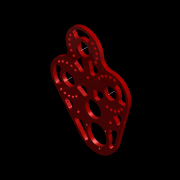
# Autodesk Inventor part: Part2
Saved by Autodesk Inventor 2014 SP1 (Build 180222100, 222)
## iProperties
Created: 2014-01-05
Part Number: Part2
Material: Aluminum 6061
Document SubType Name: Modeling
Designer: Rauhul Varma
Density: 2.71 g/cm^3
Appearance: Red
Mass: 189.365 g
Surface Area: 361.578 cm^2
Volume: 69.8764 cm^3
Author: Rauhul Varma
Autodesk Inventor part; units mm, degrees
note: some values were not read from the file. Chosen so that the rebuilt part matches the saved one: direction of "Hole3".
ref_plane "YZ Plane" through (0, 0, 0) normal (1, 0, 0) x (0, 1, 0)
ref_plane "XZ Plane" through (0, 0, 0) normal (0, 1, 0) x (-1, 0, 0)
sketch "Main Outline" plane through (0, 0, 0) normal (0, 0, 1) x (1, 0, 0)
  line L0 (0, 0) -> (304.8, 0) construction
  line L1 (304.8, 0) -> (304.8, 50.8) construction
  line L2 (304.8, 50.8) -> (0, 50.8) construction
  line L3 (0, 50.8) -> (0, 0) construction
  line L4 (0, 50.8) -> (0, 53.34) construction
  line L5 (0, 53.34) -> (304.8, 53.34) construction
  line L6 (304.8, 53.34) -> (304.8, 50.8) construction
  circle A0 centre (152.4, 23.8125) radius 17.4625 construction
  line L7 (152.4, 23.8125) -> (152.4, 0) construction
  circle A1 centre (152.4, 23.8125) radius 27.94 construction
  circle A2 centre (152.4, 23.8125) radius 21.59 construction
  line L8 (152.4, 23.8125) -> (144.7964, 60.3681) construction
  circle A3 centre (144.7964, 60.3681) radius 15.24 construction
  circle A4 centre (144.7964, 60.3681) radius 8.89 construction
  circle A5 centre (144.7964, 60.3681) radius 14.2875 construction
  arc A6 (164.6591, 71.8014) -> (129.0153, 43.7486) centre (144.7964, 60.3681) ccw construction
  circle A7 centre (98.8106, 85.598) radius 32.258 construction
  circle A8 centre (126.6733, 147.4971) radius 32.258 construction
  circle A9 centre (176.9075, 101.8424) radius 32.258 construction
  circle A10 centre (144.7964, 60.3681) radius 11.1125 construction
  circle A11 centre (152.4, 23.8125) radius 49.53 construction
  line L9 (144.7964, 60.3681) -> (126.6733, 147.4971) construction
  line L10 (144.7964, 60.3681) -> (98.8106, 85.598) construction
  line L11 (98.8106, 85.598) -> (176.9075, 101.8424) construction
  line L12 (176.9075, 101.8424) -> (144.7964, 60.3681) construction
  circle A12 centre (98.8106, 85.598) radius 9.5493 construction
  arc A13 (174.9629, 111.1915) -> (185.6989, 98.1139) centre (176.9075, 101.8424) ccw construction
  circle A14 centre (126.6733, 147.4971) radius 9.5493 construction
  line L13 (96.8659, 94.9472) -> (174.9629, 111.1915) construction
  line L14 (185.6989, 98.1139) -> (165.8956, 51.4198) construction
  line L15 (92.2351, 78.6732) -> (129.0153, 43.7486) construction
  line L16 (174.9629, 111.1915) -> (176.9075, 101.8424) construction
  line L17 (176.9075, 101.8424) -> (185.6989, 98.1139) construction
  arc A15 (185.6989, 98.1139) -> (174.9629, 111.1915) centre (176.9075, 101.8424) ccw construction
  arc A16 (165.8956, 51.4198) -> (164.6591, 71.8014) centre (144.7964, 60.3681) ccw construction
  arc A17 (129.0153, 43.7486) -> (165.8956, 51.4198) centre (144.7964, 60.3681) ccw construction
  circle A18 centre (126.6086, 147.808) radius 32.258 construction
  circle A19 centre (126.544, 148.1188) radius 32.258 construction
  circle A20 centre (126.4793, 148.4297) radius 32.258 construction
  line L18 (126.6733, 147.4971) -> (126.4793, 148.4297) construction
  circle A21 centre (126.738, 147.1863) radius 32.258 construction
  circle A22 centre (117.4622, 43.2997) radius 9.525 construction
  circle A23 centre (176.6694, 55.615) radius 9.525 construction
  line L19 (152.4, 23.8125) -> (117.4622, 43.2997) construction
  line L20 (152.4, 23.8125) -> (176.6694, 55.615) construction
  line L21 (117.4622, 43.2997) -> (98.8106, 85.598) construction
  line L22 (176.6694, 55.615) -> (176.9075, 101.8424) construction
  circle A24 centre (135.1821, 106.5897) radius 7.9375 construction
  line L23 (135.6243, 150.8242) -> (166.2787, 68.353) construction
  circle A25 centre (152.4, 23.8125) radius 29.845 construction
  line L24 (117.1381, 146.979) -> (121.9118, 59.1246) construction
  circle A26 centre (99.0889, 85.4453) radius 32.258 construction
  circle A27 centre (97.9755, 86.0562) radius 32.258 construction
  line L25 (97.9755, 86.0562) -> (98.8106, 85.598) construction
  circle A28 centre (98.2538, 85.9034) radius 32.258 construction
  circle A29 centre (98.5322, 85.7507) radius 32.258 construction
  circle A30 centre (152.4, 23.8125) radius 29.845 construction
  circle A31 centre (122.555, 23.8125) radius 6.35 construction
  circle A32 centre (179.7696, 35.7133) radius 6.35 construction
  line L26 (122.555, 23.8125) -> (152.4, 23.8125) construction
  line L27 (152.4, 23.8125) -> (182.245, 23.8125) construction
  circle A33 centre (182.245, 23.8125) radius 6.35 construction
  circle A34 centre (125.0304, 11.9117) radius 6.35 construction
  circle A35 centre (150.4199, 33.3321) radius 39.5684 construction
  line L28 (72.9795, 65.6655) -> (119.7593, 8.3204) construction
  circle A36 centre (177.4906, 102.5955) radius 32.258 construction
  line L29 (176.9075, 101.8424) -> (177.4906, 102.5955) construction
  circle A37 centre (177.2963, 102.3445) radius 32.258 construction
  circle A38 centre (177.1019, 102.0934) radius 32.258 construction
  circle A39 centre (176.7131, 101.5913) radius 32.258 construction
  line L30 (188.5109, 22.6209) -> (208.5442, 93.8632) construction
  circle A40 centre (135.1821, 106.5897) radius 9.5727 construction
  arc A41 (86.8202, 116.3239) -> (96.3065, 136.4856) centre (81.3304, 131.2195) ccw construction
  arc A42 (158.9123, 149.5077) -> (175.6513, 134.801) centre (174.7462, 150.6502) ccw construction
  line L31 (126.4793, 148.4297) -> (126.9966, 145.9429) construction
  line L32 (116.5322, 146.3607) -> (117.0495, 143.8739) construction
  line L33 (136.9437, 148.0119) -> (136.4264, 150.4987) construction
  arc A43 (136.4264, 150.4987) -> (116.5322, 146.3607) centre (126.4793, 148.4297) ccw construction
  arc A44 (117.0495, 143.8739) -> (136.9437, 148.0119) centre (126.9966, 145.9429) ccw construction
  line L34 (177.4906, 102.5955) -> (175.9357, 100.5871) construction
  line L35 (169.4571, 108.8154) -> (167.9021, 106.807) construction
  line L36 (183.9692, 94.3672) -> (185.5242, 96.3756) construction
  arc A45 (185.5242, 96.3756) -> (169.4571, 108.8154) centre (177.4906, 102.5955) ccw construction
  arc A46 (167.9021, 106.807) -> (183.9692, 94.3672) centre (175.9357, 100.5871) ccw construction
  line L37 (97.9755, 86.0562) -> (100.2023, 84.8344) construction
  line L38 (93.0884, 77.1487) -> (95.3153, 75.927) construction
  line L39 (105.0894, 93.7418) -> (102.8625, 94.9636) construction
  arc A47 (102.8625, 94.9636) -> (93.0884, 77.1487) centre (97.9755, 86.0562) ccw construction
  arc A48 (95.3153, 75.927) -> (105.0894, 93.7418) centre (100.2023, 84.8344) ccw construction
  circle A49 centre (117.4622, 43.2997) radius 3.9687 construction
  circle A50 centre (176.6694, 55.615) radius 3.9687 construction
  line L40 (152.4, 23.8125) -> (158.4777, -5.4071) construction
  arc A51 (80.1751, 59.3139) -> (79.0947, 58.1692) centre (79.7097, 58.6709) ccw construction
  arc A52 (205.9254, 84.5503) -> (204.4781, 85.1692) centre (205.1613, 84.7652) ccw construction
  circle A53 centre (152.4, 23.8125) radius 14.224 construction
  circle A54 centre (135.1821, 106.5897) radius 3.9687 construction
  circle A55 centre (156.538, 3.9183) radius 6.35 construction
  circle A56 centre (156.538, 3.9183) radius 2.0828 construction
  circle A57 centre (152.4, 23.8125) radius 20.32 construction
  line L41 (133.1021, 30.1759) -> (152.4, 23.8125) construction
  line L42 (152.4, 23.8125) -> (167.5599, 37.3432) construction
  circle A58 centre (167.5599, 37.3432) radius 2.0828 construction
  circle A59 centre (167.5599, 37.3432) radius 3.9687 construction
  circle A60 centre (133.1021, 30.1759) radius 2.0828 construction
  circle A61 centre (133.1021, 30.1759) radius 3.9688 construction
  point P0 (126.738, 147.1863)
  point P1 (176.7131, 101.5913)
  dimension "d18" = 99.06
  dimension "d58" = 64.516
  dimension "d86" = 64.516
  dimension "d0" = 304.8
  dimension "d1" = 50.8
  dimension "d2" = 2.54
  dimension "d3" = 34.925
  dimension "d4" = 23.8125
  dimension "d5" = 152.4
  dimension "d6" = 55.88
  dimension "d7" = 43.18
  dimension "d8" = 37.338
  dimension "d10" = 30.48
  dimension "d11" = 17.78
  dimension "d12" = 28.575
  dimension "d13" = 45.8366
  dimension "d14" = 64.516
  dimension "d15" = 64.516
  dimension "d16" = 64.516
  dimension "d17" = 22.225
  dimension "d19" = 52.4523
  dimension "d20" = 88.9939
  dimension "d21" = 19.0986
  dimension "d22" = 19.0986
  dimension "d23" = 19.0986
  dimension "d30" = 124.732
  dimension "d40" = 64.516
  dimension "d41" = 64.516
  dimension "d42" = 64.516
  dimension "d43" = 0.9525
  dimension "d44" = 0.3175
  dimension "d45" = 0.635
  dimension "d46" = 64.516
  dimension "d47" = 0.3175
  dimension "d48" = 19.05
  dimension "d49" = 19.05
  dimension "d50" = 40.005
  dimension "d51" = 40.005
  dimension "d52" = 46.228
  dimension "d54" = 46.228
  dimension "d55" = 15.875
  dimension "d56" = 41.4655
  dimension "d57" = 59.69
  dimension "d59" = 64.516
  dimension "d60" = 64.516
  dimension "d61" = 64.516
  dimension "d62" = 0.3175
  dimension "d63" = 0.3175
  dimension "d64" = 0.635
  dimension "d65" = 0.9525
  dimension "d73" = 12.7
  dimension "d74" = 12.7
  dimension "d76" = 59.69
  dimension "d78" = 12.7
  dimension "d79" = 12.7
  dimension "d80" = 64.516
  dimension "d81" = 0.9525
  dimension "d82" = 64.516
  dimension "d83" = 64.516
  dimension "d84" = 0.3175
  dimension "d85" = 0.635
  dimension "d88" = 0.3175
  dimension "d89" = 31.75
  dimension "d90" = 31.75
  dimension "d94" = 1.5875
  dimension "d95" = 20.32
  dimension "d96" = 1.5875
  constraints: 92 end point, 59 centre point, 54 point on circle, 38 tangent, 26 coincident, 16 point on line, 9 collinear, 6 parallel, 4 midpoint, 4 perpendicular, 3 symmetric about line, 2 horizontal, 13 other
  measures "d0" distance of L2.end L1.end
  measures "d1" distance of L1.end L0.end
  measures "d2" distance of L2.end L4.end
  measures "d3" diameter of A0
  measures "d4" distance of L7.start L7.end
  measures "d5" distance between parallel lines of L3 L7
  measures "d6" diameter of A1
  measures "d7" diameter of A2
  measures "d8" distance of L8.start L8.end
  measures "d10" diameter of A3
  measures "d11" diameter of A4
  measures "d12" diameter of A5
  measures "d13" diameter of A6
  measures "d14" diameter of A7
  measures "d15" diameter of A8
  measures "d16" diameter of A9
  measures "d17" diameter of A10
  measures "d19" distance of L9.start L10.end
  measures "d20" distance of L9.start L9.end
  measures "d21" diameter of A12
  measures "d22" diameter of A13
  measures "d23" diameter of A14
  measures "d30" angle of L17 L16
  measures "d40" diameter of A18
  measures "d41" diameter of A19
  measures "d42" diameter of A20
  measures "d43" distance of L18.end L9.end
  measures "d44" distance of A18.centre L9.end
  measures "d45" distance of A19.centre L9.end
  measures "d46" diameter of A21
  measures "d47" distance of L9.end A21.centre
  measures "d48" diameter of A22
  measures "d49" diameter of A23
  measures "d50" distance of L19.start L19.end
  measures "d51" distance of L19.start L20.end
  measures "d52" distance of L19.end L21.end
  measures "d54" distance of L20.end L16.end
  measures "d55" diameter of A24
  measures "d56" distance of A21.centre A24.centre
  measures "d57" diameter of A25
  measures "d59" diameter of A27
  measures "d60" diameter of A28
  measures "d61" diameter of A29
  measures "d62" distance of point (99.089, 85.445) L10.end
  measures "d63" distance of L10.end A29.centre
  measures "d64" distance of L10.end A28.centre
  measures "d65" distance of L25.start L10.end
  measures "d73" diameter of A31
  measures "d74" diameter of A32
  measures "d76" diameter of A30
  measures "d78" diameter of A33
  measures "d79" diameter of A34
  measures "d80" diameter of A36
  measures "d81" distance of L29.start L29.end
  measures "d82" diameter of A37
  measures "d83" diameter of A38
  measures "d84" distance of L16.end A38.centre
  measures "d85" distance of L11.end A37.centre
  measures "d88" distance of L11.end point (176.713, 101.591)
  measures "d89" diameter of A41
  measures "d90" diameter of A42
  measures "d94" distance of L9.end L31.end
  measures "d95" diameter of A44
  measures "d96" distance of L11.end L34.end
sketch "Upper CIM C-C Check" plane through (0, 0, 0) normal (0, 0, 1) x (1, 0, 0)
  arc A0 (3.4429, -22.6582) -> (3.4429, 22.6582) centre (0, 0) ccw construction
  arc A1 (90.4285, 9.4409) -> (90.4285, -9.4409) centre (88.9939, 0) ccw construction
  line L0 (88.9939, 0) -> (0, 0) construction
  line L1 (90.4285, 9.4409) -> (3.4429, 22.6582)
  line L2 (3.4429, -22.6582) -> (90.4285, -9.4409)
  arc A2 (90.4285, -9.4409) -> (90.4285, 9.4409) centre (88.9939, 0) ccw
  arc A3 (3.4429, 22.6582) -> (3.4429, -22.6582) centre (0, 0) ccw
  dimension "d24" = 45.8366
  dimension "d25" = 19.0986
  dimension "d26" = 78.9119
  dimension "d27" = 87.984
  dimension "d28" = 27.12
  dimension "d29" = 88.9939
  constraints: 8 point on circle, 6 end point, 4 centre point, 4 tangent, 1 coincident, 1 horizontal
  measures "d24" diameter of A0
  measures "d25" diameter of A1
  measures "d27" distance of L1.start L1.end
  measures "d29" distance of L0.start L0.end
sketch "Motor Plate" plane through (0, 0, 0) normal (0, 0, 1) x (1, 0, 0)
  arc A0 (158.9123, 149.5077) -> (175.6513, 134.801) centre (174.7462, 150.6502) ccw projected
  arc A1 (86.8202, 116.3239) -> (96.3065, 136.4856) centre (81.3304, 131.2195) ccw projected
  circle A2 centre (97.9755, 86.0562) radius 32.258 projected
  line L0 (72.9795, 65.6655) -> (119.7593, 8.3204) projected
  circle A3 centre (150.4199, 33.3321) radius 39.5684 projected
  line L1 (188.5109, 22.6209) -> (208.5442, 93.8632) projected
  circle A4 centre (177.4906, 102.5955) radius 32.258 projected
  circle A5 centre (144.7964, 60.3681) radius 14.2875 projected
  circle A6 centre (135.1821, 106.5897) radius 7.9375 construction
  circle A7 centre (117.4622, 43.2997) radius 9.525 construction
  circle A8 centre (176.6694, 55.615) radius 9.525 construction
  arc A9 (136.4264, 150.4987) -> (116.5322, 146.3607) centre (126.4793, 148.4297) ccw projected
  arc A10 (117.0495, 143.8739) -> (136.9437, 148.0119) centre (126.9966, 145.9429) ccw projected
  line L2 (116.5322, 146.3607) -> (117.0495, 143.8739) projected
  line L3 (136.9437, 148.0119) -> (136.4264, 150.4987) projected
  arc A11 (185.5242, 96.3756) -> (169.4571, 108.8154) centre (177.4906, 102.5955) ccw projected
  arc A12 (167.9021, 106.807) -> (183.9692, 94.3672) centre (175.9357, 100.5871) ccw projected
  line L4 (183.9692, 94.3672) -> (185.5242, 96.3756) projected
  arc A13 (102.8625, 94.9636) -> (93.0884, 77.1487) centre (97.9755, 86.0562) ccw projected
  arc A14 (95.3153, 75.927) -> (105.0894, 93.7418) centre (100.2023, 84.8344) ccw projected
  line L5 (105.0894, 93.7418) -> (102.8625, 94.9636) projected
  line L6 (93.0884, 77.1487) -> (95.3153, 75.927) projected
  line L7 (169.4571, 108.8154) -> (167.9021, 106.807) projected
  circle A15 centre (152.4, 23.8125) radius 17.4625 projected
  circle A16 centre (167.5599, 37.3432) radius 2.0828 construction
  circle A17 centre (156.538, 3.9183) radius 2.0828 construction
  circle A18 centre (133.1021, 30.1759) radius 2.0828 construction
  line L8 (126.4793, 148.4297) -> (144.7964, 60.3681) construction
  line L9 (144.7964, 60.3681) -> (177.4906, 102.5955) construction
  line L10 (144.7964, 60.3681) -> (97.9755, 86.0562) construction
  circle A19 centre (126.738, 147.1863) radius 32.258 projected
  line L11 (92.7728, 60.926) -> (104.8483, 110.27) construction
  line L12 (85.9116, 63.7308) -> (112.2662, 107.1598) construction
  line L13 (96.8659, 94.9472) -> (174.9629, 111.1915) construction
  line L14 (92.2351, 78.6732) -> (129.0153, 43.7486) construction
  line L15 (185.6989, 98.1139) -> (165.8956, 51.4198) construction
  line L16 (117.1381, 146.979) -> (121.9118, 59.1246) construction
  line L17 (135.6243, 150.8242) -> (166.2787, 68.353) construction
  line L18 (100.1929, 60.4051) -> (96.8715, 111.0964) construction
  line L19 (107.4593, 62.2302) -> (89.0484, 109.5766) construction
  line L20 (113.8735, 66.2468) -> (82.0774, 105.8656) construction
  circle A20 centre (126.4793, 148.4297) radius 32.258 projected
  line L21 (158.0614, 154.9988) -> (158.32, 153.7554)
  line L22 (94.8973, 141.8606) -> (95.1559, 140.6172)
  line L23 (104.5119, 135.0861) -> (148.8347, 159.9082) construction
  line L24 (109.3343, 128.6856) -> (144.1416, 165.687) construction
  line L25 (101.7409, 142.6354) -> (151.4764, 152.9805) construction
  line L26 (101.2718, 150.6636) -> (151.8162, 145.5741) construction
  line L27 (103.142, 158.4561) -> (149.8166, 138.4032) construction
  point P0 (0, 0)
  point P1 (98.2538, 85.9034)
  point P2 (98.5322, 85.7507)
  point P3 (98.8106, 85.598)
  point P4 (99.0889, 85.4453)
  point P5 (161.5326, 122.0604)
  point P6 (192.2825, 81.6243)
  point P7 (155.9701, 116.2503)
  point P8 (197.4562, 86.9323)
  point P9 (170.8103, 78.0897)
  point P10 (178.2941, 76.9641)
  point P11 (176.2984, 127.7248)
  point P12 (184.171, 127.1013)
  point P13 (168.5182, 125.9991)
  point P14 (185.6856, 78.1877)
  point P15 (126.6733, 147.4971)
  point P16 (126.738, 147.1863)
  point P17 (126.544, 148.1188)
  point P18 (126.6086, 147.808)
  dimension "d119" = 0.3175
  dimension "d120" = 0.3175
  dimension "d121" = 0.3175
  dimension "d122" = 0.3175
  dimension "d124" = 50.8
  dimension "d125" = 50.8
  dimension "d126" = 87.5
  dimension "d127" = 25.4
  dimension "d128" = 122.5
  dimension "d129" = 50.8
  dimension "d130" = 25.4
  dimension "d131" = 50.8
  dimension "d132" = 25.4
  dimension "d133" = 140
  dimension "d134" = 157.5
  dimension "d135" = 50.8
  dimension "d136" = 25.4
  dimension "d145" = 105
  dimension "d146" = 25.4
  dimension "d147" = 0.3175
  dimension "d148" = 0.3175
  dimension "d149" = 0.3175
  dimension "d150" = 0.3175
  dimension "d151" = 107.5
  dimension "d152" = 125
  dimension "d153" = 90
  dimension "d154" = 50.8
  dimension "d155" = 50.8
  dimension "d156" = 50.8
  dimension "d157" = 25.4
  dimension "d158" = 25.4
  dimension "d159" = 25.4
  dimension "d160" = 50.8
  dimension "d161" = 50.8
  dimension "d162" = 25.4
  dimension "d163" = 72.5
  dimension "d164" = 55
  constraints: 30 end point, 27 coincident, 10 midpoint, 10 symmetric about line, 8 point on line, 4 point on circle, 4 tangent, 3 parallel
  measures "d119" distance of A2.centre point (98.254, 85.903)
  measures "d120" distance of point (98.254, 85.903) point (98.532, 85.751)
  measures "d121" distance of point (98.532, 85.751) point (98.811, 85.598)
  measures "d122" distance of point (98.811, 85.598) point (99.089, 85.445)
  measures "d124" distance of L11.start L11.end
  measures "d125" distance of L12.start L12.end
  measures "d126" angle of L12 L10
  measures "d127" distance of point (99.089, 85.445) L12.end
  measures "d128" angle of L10 L18
  measures "d129" distance of L18.start L18.end
  measures "d130" distance of L18.end point (98.532, 85.751)
  measures "d131" distance of L19.start L19.end
  measures "d132" distance of point (98.254, 85.903) L19.start
  measures "d133" angle of L10 L19
  measures "d134" angle of L10 L20
  measures "d135" distance of L20.start L20.end
  measures "d136" distance of A2.centre L20.start
  measures "d145" angle of L10 L11
  measures "d146" distance of point (98.811, 85.598) L11.end
  measures "d147" distance of L8.start point (126.544, 148.119)
  measures "d148" distance of point (126.544, 148.119) point (126.609, 147.808)
  measures "d149" distance of point (126.609, 147.808) point (126.673, 147.497)
  measures "d150" distance of point (126.673, 147.497) point (126.738, 147.186)
  measures "d151" angle of L8 L23
  measures "d152" angle of L8 L24
  measures "d153" angle of L8 L25
  measures "d154" distance of L23.start L23.end
  measures "d155" distance of L24.start L24.end
  measures "d156" distance of L25.start L25.end
  measures "d157" distance of point (126.738, 147.186) L24.end
  measures "d158" distance of point (126.673, 147.497) L23.end
  measures "d159" distance of point (126.609, 147.808) L25.end
  measures "d160" distance of L27.start L27.end
  measures "d161" distance of L26.start L26.end
  measures "d162" distance of L26.start point (126.544, 148.119)
  measures "d163" angle of L8 L26
  measures "d164" angle of L8 L27
extrude "Profile" add sketch "Motor Plate" along normal blind 6.35 contours A0 A4 L1 A3 A5 L0 A2 A1 A19 | A19 A20 | A4 | A19 A20 L21 | A20 A19 | A19 A20 | A3 A5 | A2 | L22 A20 A19 | A5 A3 | A3 A5 | L3 A10 L2 A9 | L4 A12 L7 A11 | L5 A14 L6 A13 | A15
extrude "Bearing and Motor Cutouts" cut sketch "Motor Plate" along normal through all contours A5 A3 | A3 A5 | L3 A10 L2 A9 | L4 A12 L7 A11 | L5 A14 L6 A13 | A15 picked at (142.2205, 72.7522) picked at (143.8851, 63.378)
hole "10-32 Clearance Holes" at (135.1821, 106.5897, 0) at (117.4622, 43.2997, 0) at (176.6694, 55.615, 0) at (104.8483, 110.27, 0) at (92.7728, 60.926, 0) at (112.2662, 107.1598, 0) at (85.9116, 63.7308, 0) at (113.8735, 66.2468, 0) at (107.4593, 62.2302, 0) at (89.0484, 109.5766, 0) at (82.0774, 105.8656, 0) at (96.8715, 111.0964, 0) at (100.1929, 60.4051, 0) at (161.5326, 122.0604, 0) at (155.9701, 116.2503, 0) at (168.5182, 125.9991, 0) at (176.2984, 127.7248, 0) at (184.171, 127.1013, 0) at (197.4562, 86.9323, 0) at (192.2825, 81.6243, 0) at (185.6856, 78.1877, 0) at (178.2941, 76.9641, 0) at (170.8103, 78.0897, 0) at (109.3343, 128.6856, 0) at (104.5119, 135.0861, 0) at (101.7409, 142.6354, 0) at (101.2718, 150.6636, 0) at (103.142, 158.4561, 0) at (144.1416, 165.687, 0) at (148.8347, 159.9082, 0) at (151.4764, 152.9805, 0) at (151.8162, 145.5741, 0) at (149.8166, 138.4032, 0) direction (0, 0, 1) diameter 4.9784 end through all clearance for "Socket Head Cap Screw" size "#10" standard "Ansi Unified Screw Threads"
hole "Hole2" at (167.5599, 37.3432, 0) at (133.1021, 30.1759, 0) at (156.538, 3.9183, 0) direction (0, 0, 1) diameter 3.302 end through all thread size "8-32 UNC" class "2B" standard "ANSI Unified Screw Threads"
ref_plane "Work Plane1" through (152.4, 23.8125, 0) normal (0.9790451, 0.2036437, 0) x (-0.2036437, 0.9790451, 0)
sketch "Sketch5" plane through (0, 0, 6.35) normal (0, 0, 1) x (1, 0, 0)
  circle A0 centre (167.5599, 37.3432) radius 1.651 projected
  circle A1 centre (178.2941, 76.9641) radius 2.4892 projected
  circle A2 centre (192.2825, 81.6243) radius 2.4892 projected
  circle A3 centre (184.171, 127.1013) radius 2.4892 projected
  circle A4 centre (135.1821, 106.5897) radius 2.4892 projected
  circle A5 centre (176.6694, 55.615) radius 2.4892 projected
  circle A6 centre (155.9701, 116.2503) radius 2.4892 projected
  circle A7 centre (197.4562, 86.9323) radius 2.4892 projected
  circle A8 centre (185.6856, 78.1877) radius 2.4892 projected
  circle A9 centre (170.8103, 78.0897) radius 2.4892 projected
  circle A10 centre (149.8166, 138.4032) radius 2.4892 projected
  circle A11 centre (152.4, 23.8125) radius 17.4625 projected
  line L0 (95.3153, 75.927) -> (93.0884, 77.1487) projected
  circle A12 centre (144.7964, 60.3681) radius 14.2875 projected
  line L1 (185.5242, 96.3756) -> (183.9692, 94.3672) projected
  arc A13 (167.9021, 106.807) -> (183.9692, 94.3672) centre (175.9357, 100.5871) ccw projected
  line L2 (167.9021, 106.807) -> (169.4571, 108.8154) projected
  arc A14 (185.5242, 96.3756) -> (169.4571, 108.8154) centre (177.4906, 102.5955) ccw projected
  line L3 (136.4264, 150.4987) -> (136.9437, 148.0119) projected
  arc A15 (117.0495, 143.8739) -> (136.9437, 148.0119) centre (126.9966, 145.9429) ccw projected
  line L4 (117.0495, 143.8739) -> (116.5322, 146.3607) projected
  arc A16 (136.4264, 150.4987) -> (116.5322, 146.3607) centre (126.4793, 148.4297) ccw projected
  arc A17 (158.9123, 149.5077) -> (158.32, 153.7554) centre (126.738, 147.1863) ccw projected
  line L5 (158.32, 153.7554) -> (158.0614, 154.9988) projected
  arc A18 (158.0614, 154.9988) -> (94.8973, 141.8606) centre (126.4793, 148.4297) ccw projected
  line L6 (94.8973, 141.8606) -> (95.1559, 140.6172) projected
  arc A19 (95.1559, 140.6172) -> (96.3065, 136.4856) centre (126.738, 147.1863) ccw projected
  arc A20 (86.8202, 116.3239) -> (96.3065, 136.4856) centre (81.3304, 131.2195) ccw projected
  arc A21 (86.8202, 116.3239) -> (72.9795, 65.6655) centre (97.9755, 86.0562) ccw projected
  line L7 (72.9795, 65.6655) -> (119.7593, 8.3204) projected
  arc A22 (119.7593, 8.3204) -> (188.5109, 22.6209) centre (150.4199, 33.3321) ccw projected
  line L8 (188.5109, 22.6209) -> (208.5442, 93.8632) projected
  arc A23 (208.5442, 93.8632) -> (175.6513, 134.801) centre (177.4906, 102.5955) ccw projected
  arc A24 (158.9123, 149.5077) -> (175.6513, 134.801) centre (174.7462, 150.6502) ccw projected
  line L9 (97.9755, 86.0562) -> (177.4906, 102.5955) construction
  line L10 (152.4, 23.8125) -> (126.4793, 148.4297) construction
  line L11 (97.9755, 86.0562) -> (144.7964, 60.3681) construction
  line L12 (177.4906, 102.5955) -> (144.7964, 60.3681) construction
  line L13 (169.7116, 97.7345) -> (107.0476, 84.7002) construction
  line L14 (107.0476, 84.7002) -> (143.946, 64.4561) construction
  line L15 (143.946, 64.4561) -> (169.7116, 97.7345) construction
  line L16 (185.2696, 107.4565) -> (88.9033, 87.4121) construction
  line L17 (88.9033, 87.4121) -> (145.6467, 56.2801) construction
  line L18 (145.6467, 56.2801) -> (185.2696, 107.4565) construction
  line L19 (146.2021, 22.4281) -> (120.2814, 147.0453) construction
  line L20 (158.8075, 24.1896) -> (132.8868, 148.8068) construction
  line L21 (187.7349, 91.4516) -> (189.2899, 93.46) construction
  arc A25 (189.2899, 93.46) -> (165.6913, 111.731) centre (177.4906, 102.5955) ccw construction
  line L22 (165.6913, 111.731) -> (164.1364, 109.7226) construction
  arc A26 (164.1364, 109.7226) -> (187.7349, 91.4516) centre (175.9357, 100.5871) ccw construction
  circle A27 centre (144.7964, 60.3681) radius 19.05 construction
  circle A28 centre (135.1821, 106.5897) radius 7.9375 construction
  circle A29 centre (155.9701, 116.2503) radius 7.2517 construction
  circle A30 centre (158.2601, 105.753) radius 3.4925 construction
  arc A31 (154.9567, 109.0697) -> (142.1051, 102.7069) centre (153.1819, 96.4944) ccw construction
  circle A32 centre (146.6588, 102.9926) radius 3.4925 construction
  circle A33 centre (149.8166, 138.4032) radius 7.2517 construction
  line L23 (141.6064, 148.9818) -> (141.0891, 151.4686) construction
  arc A34 (141.0891, 151.4686) -> (111.8695, 145.3908) centre (126.4793, 148.4297) ccw construction
  line L24 (111.8695, 145.3908) -> (112.3868, 142.904) construction
  arc A35 (112.3868, 142.904) -> (141.6064, 148.9818) centre (126.9966, 145.9429) ccw construction
  arc A36 (143.441, 134.948) -> (137.8341, 135.6847) centre (140.3705, 133.2839) ccw construction
  arc A37 (151.6322, 122.0615) -> (149.0973, 131.1873) centre (148.5934, 126.1324) ccw construction
  arc A38 (203.9596, 95.1525) -> (175.9229, 130.0463) centre (177.4906, 102.5955) ccw construction
  line L25 (203.9596, 95.1525) -> (183.9262, 23.9101) construction
  arc A39 (123.4497, 11.3309) -> (183.9262, 23.9101) centre (150.4199, 33.3321) ccw construction
  line L26 (123.4497, 11.3309) -> (76.6699, 68.6759) construction
  arc A40 (88.4671, 111.8553) -> (76.6699, 68.6759) centre (97.9755, 86.0562) ccw construction
  arc A41 (88.4671, 111.8553) -> (100.7993, 138.0654) centre (81.3304, 131.2195) ccw construction
  arc A42 (99.8186, 141.587) -> (100.7993, 138.0654) centre (126.738, 147.1863) ccw construction
  line L27 (99.8186, 141.587) -> (99.56, 142.8304) construction
  arc A43 (153.3987, 154.029) -> (99.56, 142.8304) centre (126.4793, 148.4297) ccw construction
  line L28 (153.3987, 154.029) -> (153.6573, 152.7856) construction
  arc A44 (154.1622, 149.165) -> (153.6573, 152.7856) centre (126.738, 147.1863) ccw construction
  arc A45 (154.1622, 149.165) -> (175.9229, 130.0463) centre (174.7462, 150.6502) ccw construction
  circle A46 centre (184.171, 127.1013) radius 7.2517 construction
  circle A47 centre (197.4562, 86.9323) radius 7.2517 construction
  arc A48 (187.1433, 120.4867) -> (186.4727, 114.5121) centre (188.5748, 117.301) ccw construction
  arc A49 (191.814, 98.4094) -> (195.9106, 94.0174) centre (195.1662, 97.4297) ccw construction
  circle A50 centre (178.2941, 76.9641) radius 7.2517 construction
  circle A51 centre (176.6694, 55.615) radius 11.9062 construction
  circle A52 centre (185.6856, 78.1877) radius 7.2517 construction
  circle A53 centre (192.2825, 81.6243) radius 7.2517 construction
  arc A54 (186.23, 70.9565) -> (184.2644, 64.7842) centre (186.4922, 67.4739) ccw construction
  arc A55 (196.8445, 69.8499) -> (190.948, 73.1983) centre (193.4824, 70.7954) ccw construction
  arc A56 (187.6577, 60.1993) -> (194.243, 60.5986) centre (190.8809, 61.544) ccw construction
  circle A57 centre (170.8103, 78.0897) radius 7.2517 construction
  circle A58 centre (167.5599, 37.3432) radius 6.4135 construction
  circle A59 centre (152.4, 23.8125) radius 22.225 construction
  arc A60 (176.955, 43.7121) -> (173.6968, 39.2062) centre (177.0388, 40.2206) ccw construction
  arc A61 (189.0701, 42.2026) -> (183.658, 45.9756) centre (185.708, 43.148) ccw construction
  arc A62 (173.8743, 18.0848) -> (180.2411, 15.3838) centre (177.2488, 17.1848) ccw construction
  arc A63 (139.4535, 117.2365) -> (148.8152, 117.431) centre (144.1162, 118.2064) ccw construction
  arc A64 (176.955, 43.7121) -> (173.6968, 39.2062) centre (177.0388, 40.2206) ccw
  arc A65 (172.5129, 33.2689) -> (173.6968, 39.2062) centre (167.5599, 37.3432) ccw
  arc A66 (173.8743, 18.0848) -> (172.5129, 33.2689) centre (152.4, 23.8125) ccw
  arc A67 (176.955, 43.7121) -> (183.658, 45.9756) centre (176.6694, 55.615) ccw
  arc A68 (189.0701, 42.2026) -> (183.658, 45.9756) centre (185.708, 43.148) ccw
  arc A69 (173.8743, 18.0848) -> (180.2411, 15.3838) centre (177.2488, 17.1848) ccw
  arc A70 (180.2411, 15.3838) -> (183.9262, 23.9101) centre (150.4199, 33.3321) ccw
  line L29 (183.9262, 23.9101) -> (189.0701, 42.2026)
  arc A71 (186.23, 70.9565) -> (184.2644, 64.7842) centre (186.4922, 67.4739) ccw
  arc A72 (187.6577, 60.1993) -> (184.2644, 64.7842) centre (176.6694, 55.615) ccw
  arc A73 (187.6577, 60.1993) -> (194.243, 60.5986) centre (190.8809, 61.544) ccw
  arc A74 (196.8445, 69.8499) -> (190.948, 73.1983) centre (193.4824, 70.7954) ccw
  arc A75 (186.23, 70.9565) -> (190.948, 73.1983) centre (185.6856, 78.1877) ccw
  line L30 (194.243, 60.5986) -> (196.8445, 69.8499)
  line L31 (161.713, 96.0708) -> (144.5966, 92.5105)
  line L32 (144.5966, 92.5105) -> (147.3557, 79.2454)
  line L33 (153.7851, 77.1641) -> (164.4988, 91.0017)
  arc A76 (161.713, 96.0708) -> (164.4988, 91.0017) centre (175.9357, 100.5871) ccw
  arc A77 (153.7851, 77.1641) -> (147.3557, 79.2454) centre (144.7964, 60.3681) ccw
  arc A78 (144.1845, 105.4575) -> (147.37, 99.5733) centre (146.6588, 102.9926) ccw
  arc A79 (154.9567, 109.0697) -> (157.5157, 109.1652) centre (155.9701, 116.2503) ccw
  arc A80 (154.9567, 109.0697) -> (144.1845, 105.4575) centre (153.1819, 96.4944) ccw
  line L34 (147.37, 99.5733) -> (161.128, 102.435)
  arc A81 (161.6123, 104.7732) -> (157.5157, 109.1652) centre (158.2601, 105.753) ccw
  arc A82 (161.6123, 104.7732) -> (161.128, 102.435) centre (175.9357, 100.5871) ccw
  line L35 (135.9635, 134.015) -> (139.4535, 117.2365)
  arc A83 (139.4535, 117.2365) -> (148.8152, 117.431) centre (144.1162, 118.2064) ccw
  arc A84 (151.6322, 122.0615) -> (148.8152, 117.431) centre (155.9701, 116.2503) ccw
  arc A85 (151.6322, 122.0615) -> (149.0973, 131.1873) centre (148.5934, 126.1324) ccw
  arc A86 (143.441, 134.948) -> (149.0973, 131.1873) centre (149.8166, 138.4032) ccw
  arc A87 (143.441, 134.948) -> (137.8341, 135.6847) centre (140.3705, 133.2839) ccw
  arc A88 (135.9635, 134.015) -> (137.8341, 135.6847) centre (126.9966, 145.9429) ccw
  arc A89 (187.1433, 120.4867) -> (186.4727, 114.5121) centre (188.5748, 117.301) ccw
  arc A90 (188.0409, 120.9685) -> (191.381, 126.3244) centre (184.171, 127.1013) ccw
  arc A91 (203.9596, 95.1525) -> (191.381, 126.3244) centre (177.4906, 102.5955) ccw
  arc A92 (191.814, 98.4094) -> (195.9106, 94.0174) centre (195.1662, 97.4297) ccw
  arc A93 (191.814, 98.4094) -> (186.4727, 114.5121) centre (177.4906, 102.5955) ccw
  line L36 (202.9719, 91.6402) -> (203.9596, 95.1525)
  arc A94 (202.9719, 91.6402) -> (195.9106, 94.0174) centre (197.4562, 86.9323) ccw
  arc A95 (187.1433, 120.4867) -> (188.0409, 120.9685) centre (184.171, 127.1013) ccw
  circle A96 centre (103.142, 158.4561) radius 2.4892 projected
  circle A97 centre (144.1416, 165.687) radius 2.4892 projected
  circle A98 centre (103.142, 158.4561) radius 7.2517 construction
  circle A99 centre (144.1416, 165.687) radius 7.2517 construction
  arc A100 (110.1059, 160.4788) -> (115.929, 158.983) centre (113.4598, 161.4529) ccw construction
  arc A101 (132.0867, 162.2586) -> (136.891, 165.5575) centre (133.3991, 165.4951) ccw construction
  arc A102 (110.1059, 160.4788) -> (115.929, 158.983) centre (113.4598, 161.4529) ccw
  arc A103 (132.0867, 162.2586) -> (115.929, 158.983) centre (126.4793, 148.4297) ccw
  arc A104 (132.0867, 162.2586) -> (136.891, 165.5575) centre (133.3991, 165.4951) ccw
  arc A105 (140.6062, 172.0185) -> (136.891, 165.5575) centre (144.1416, 165.687) ccw
  arc A106 (110.1059, 160.4788) -> (104.9149, 165.4878) centre (103.142, 158.4561) ccw
  arc A107 (140.6062, 172.0185) -> (104.9149, 165.4878) centre (126.4793, 148.4297) ccw
  point P0 (0, 0)
  dimension "d195" = 15.875
  dimension "d196" = 6.985
  dimension "d189" = 3.175
  dimension "d191" = 4.7625
  dimension "d192" = 4.7625
  dimension "d194" = 4.7625
  dimension "d197" = 12.7
  dimension "d198" = 6.985
  dimension "d199" = 4.7625
  dimension "d200" = 4.7625
  dimension "d201" = 6.985
  dimension "d203" = 10.16
  dimension "d204" = 4.7625
  dimension "d205" = 4.7625
  dimension "d206" = 4.7625
  dimension "d207" = 6.985
  dimension "d208" = 6.985
  dimension "d209" = 4.7625
  dimension "d210" = 23.8125
  dimension "d211" = 4.7625
  dimension "d212" = 4.7625
  dimension "d213" = 6.985
  dimension "d214" = 6.985
  dimension "d215" = 6.985
  dimension "d216" = 4.7625
  dimension "d217" = 4.7625
  dimension "d218" = 4.7625
  dimension "d219" = 6.985
  dimension "d220" = 6.985
  dimension "d221" = 6.985
  dimension "d223" = 9.525
  dimension "d228" = 4.7625
  dimension "d229" = 4.7625
  dimension "d230" = 6.985
  dimension "d231" = 6.985
  dimension "d234" = 6.35
  constraints: 170 point on circle, 78 centre point, 56 end point, 48 coincident, 39 tangent, 15 point on line, 4 parallel, 3 collinear, 2 perpendicular, 36 other
  measures "d189" distance between parallel lines of L13 L9
  measures "d191" radial gap between concentric circles of A13 A26
  measures "d192" radial gap between concentric circles of A12 A27
  measures "d194" radial gap between concentric circles of A29 A6
  measures "d197" radius of A31
  measures "d198" diameter of A32
  measures "d199" radial gap between concentric circles of A10 A33
  measures "d200" radial gap between concentric circles of A15 A35
  measures "d201" diameter of A36
  measures "d203" diameter of A37
  measures "d204" radial gap between concentric circles of A23 A38
  measures "d205" radial gap between concentric circles of A3 A46
  measures "d206" radial gap between concentric circles of A47 A7
  measures "d207" diameter of A48
  measures "d208" diameter of A49
  measures "d209" radial gap between concentric circles of A1 A50
  measures "d210" diameter of A51
  measures "d211" radial gap between concentric circles of A8 A52
  measures "d212" radial gap between concentric circles of A2 A53
  measures "d213" diameter of A54
  measures "d214" diameter of A55
  measures "d215" diameter of A56
  measures "d216" radial gap between concentric circles of A9 A57
  measures "d217" radial gap between concentric circles of A58 A0
  measures "d218" radial gap between concentric circles of A11 A59
  measures "d219" diameter of A60
  measures "d220" diameter of A61
  measures "d221" diameter of A62
  measures "d223" diameter of A63
  measures "d228" radial gap between concentric circles of A96 A98
  measures "d230" diameter of A101
  measures "d231" diameter of A100
  measures "d234" distance between parallel lines of L10 L19
extrude "Extrusion3" cut sketch "Sketch5" against normal through all contours A67 A68 L29 A70 A69 A66 A65 A64 | A75 A74 L30 A73 A72 A71 | A76 L33 A77 L32 L31 | A88 A87 A86 A85 A84 A83 L35 | A95 A90 A91 L36 A94 A92 A93 A89
sketch "Sketch4" plane through (208.5442, 93.8632, 6.35) normal (0.9626636, -0.2707007, 0) x (0, 0, -1)
  line L0 (6.35, -74.0054) -> (6.35, 0) projected
  point P0 (6.35, -146.8118)
  point P1 (6.35, -9.6741)
  point P2 (3.175, -28.7241)
  dimension "d180" = 19.05
  dimension "d181" = 3.175
  measures "d180" vertical distance of point (3.175, -28.724) point (6.35, -9.674)
  measures "d181" distance from line of L0 point (3.175, -28.724)
hole "Hole3" at (200.7686, 66.2116, 3.175) direction (-0.9626636, 0.2707007, 0) diameter 2.159 end up to surface
mirror "Mirror1" about plane through (152.4, 23.8125, 0) normal (0.9790451, 0.2036437, 0) of "Extrusion3", "Hole3"
extrude "Extrusion4" cut sketch "Sketch5" against normal through all contours A106 A107 A105 A104 A103 A102
fillet "Fillet1" radius 3.175 20 edges at (135.9635, 134.015, 3.175) (172.5129, 33.2689, 3.175) (147.3557, 79.2454, 3.175) (153.7851, 77.1641, 3.175) (144.5966, 92.5105, 3.175) (161.713, 96.0708, 3.175) (164.4988, 91.0017, 3.175) (191.381, 126.3244, 3.175) (202.9719, 91.6402, 3.175) (123.5297, 131.4287, 3.175) (132.1627, 89.9242, 3.175) (115.0462, 86.364, 3.175) (114.5128, 80.6045, 3.175) (129.8557, 72.1867, 3.175) (134.9219, 76.6591, 3.175) (140.6062, 172.0185, 3.175) (104.9149, 165.4878, 3.175) (75.7752, 102.2781, 3.175) (78.9761, 65.8488, 3.175) (130.1846, 24.4645, 3.175)
equation "\"d3\" = r10"
equation "\"d6\" = g44"
equation "\"d7\" = g34"
equation "\"d10\" = g24"
equation "\"d11\" = g14"
equation "\"d12\" = r8"
equation "\"d13\" = p48"
equation "\"d14\" = cim"
equation "\"d15\" = cim"
equation "\"d16\" = cim"
equation "\"d17\" = r6"
equation "\"d21\" = p20"
equation "\"d22\" = p20"
equation "\"d23\" = p20"
equation "\"d24\" = p48"
equation "\"d25\" = p20"
equation "\"d29\" = d20"
equation "\"g14\" = 17.78"
equation "\"g24\" = 30.48"
equation "\"g34\" = 43.18"
equation "\"g44\" = 55.88"
equation "\"p20\" = 19.09859"
equation "\"p48\" = 45.83662"
equation "\"r10\" = 34.925"
equation "\"r9\" = 31.75"
equation "\"r8\" = 28.575"
equation "\"r7\" = 25.4"
equation "\"r6\" = 22.225"
equation "\"r5\" = 19.05"
equation "\"r4\" = 15.875"
equation "\"r3\" = 12.7"
equation "\"cim\" = 64.516"
equation "\"act\" = 28.448"
equation "\"actL\" = 23.749"
equation "\"UpperCimCCCheck\" = 2 * d27 + d26 + d28"
equation "\"LowerBeltPathCCCheck\" = 267"
equation "\"degoff\" = 17.5deg"
body "Solid1"
